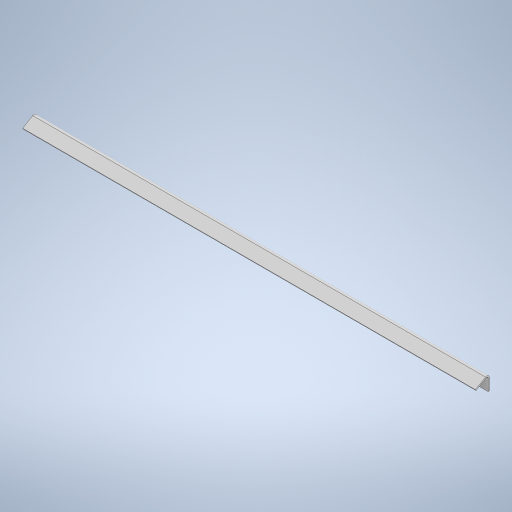
# Autodesk Inventor part: Part2
Saved by Autodesk Inventor 2023.1 (Build 271208000, 208)
## iProperties
Created: 2023-06-12
Part Number: Part2
Material: Generic
Document SubType Name: Sheet Metal
Designer: user
Density: 1 g/cm^3
Sheet Metal Rule: Default_mm
Appearance: Default
Author: user
Autodesk Inventor part; units mm, degrees
ref_plane "YZ Plane" through (0, 0, 0) normal (1, 0, 0) x (0, 1, 0)
ref_plane "XZ Plane" through (0, 0, 0) normal (0, 1, 0) x (-1, 0, 0)
ref_plane "XY Plane" through (0, 0, 0) normal (0, 0, 1) x (1, 0, 0)
sketch "Sketch1" plane through (0, 0, 0) normal (0, 0, 1) x (1, 0, 0)
  line L0 (-350, 12.5) -> (350, 12.5)
  line L1 (350, 12.5) -> (350, -12.5)
  line L2 (350, -12.5) -> (-350, -12.5)
  line L3 (-350, -12.5) -> (-350, 12.5)
  line L4 (-350, 12.5) -> (350, -12.5) construction
  line L5 (350, 12.5) -> (-350, -12.5) construction
  point P0 (0, 0)
  dimension "d0" = 700
  dimension "d1" = 25
  measures "d0" distance of L1.end L2.end
  measures "d1" distance of L0.end L1.end
extrude "Plate1" add sketch "Sketch1" along normal blind 2
sketch "Sketch2" plane through (-350, 10.7679, -1) normal (0, 0.8660254, 0.5) x (-1, 0, 0)
  line L0 (-700, 0) -> (0, 0)
  line L1 (0, 0) -> (0, 25)
  line L2 (0, 25) -> (-700, 25)
  line L3 (-700, 25) -> (-700, 0)
  constraints: 6 end point, 1 horizontal, 1 perpendicular, 1 vertical
edge flange "Flange1" height 25 angle 120 thickness 2 bend radius 2 thickness toward (0, 0.8660254, 0.5) relief straight relief width 2 relief depth 1 edges at (0, 12.5, 2) wall of the first edge with corners at (350, 10.7679, -1) (-350, 10.7679, -1) (-350, -1.7321, 20.6506) (350, -1.7321, 20.6506)
bend "Bend1"
corner "Corner1"
equation "\"d2\" = Thickness"
equation "\"d3\" = BendReliefWidth"
equation "\"d4\" = BendReliefDepth"
equation "\"d5\" = MinimumRemnant"
equation "\"d6\" = TransitionRadius"
equation "\"d9\" = BendRadius"
equation "\"d10\" = CornerReliefSize"
equation "\"d11\" = GapSize"
equation "\"d12\" = JacobiRadiusSize"
equation "\"BendRadius\" = Thickness"
equation "\"BendReliefWidth\" = Thickness"
equation "\"BendReliefDepth\" = 0.5 * Thickness"
equation "\"CornerReliefSize\" = 4 * Thickness"
equation "\"MinimumRemnant\" = 2 * Thickness"
equation "\"TransitionRadius\" = BendRadius"
equation "\"JacobiRadiusSize\" = BendRadius"
equation "\"GapSize\" = Thickness"
equation "\"Thickness\" = 2"
body "Solid1"
